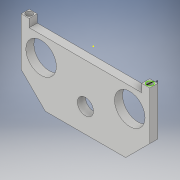
# Autodesk Inventor part: Middle_part
Saved by Autodesk Inventor 2019 (Build 230136000, 136)
## iProperties
Created: 2021-06-20
Part Number: Middle_part
Material: Generic
Document SubType Name: Modeling
Designer: 91742
Density: 1 g/cm^3
Appearance: Default
Author: 91742
Autodesk Inventor part; units mm, degrees
ref_plane "YZ Plane" through (0, 0, 0) normal (1, 0, 0) x (0, 1, 0)
ref_plane "XZ Plane" through (0, 0, 0) normal (0, 1, 0) x (-1, 0, 0)
ref_plane "XY Plane" through (0, 0, 0) normal (0, 0, 1) x (1, 0, 0)
sketch "Sketch1" plane through (0, 0, 0) normal (0, 0, 1) x (1, 0, 0)
  line L0 (-40, 5) -> (40, 5)
  circle A0 centre (-27.6, 32.5) radius 9.5
  line L1 (-40, 5) -> (-40, 50)
  line L2 (-40, 50) -> (-35, 50)
  line L3 (-35, 50) -> (-35, 45)
  line L4 (-35, 45) -> (0, 45)
  circle A1 centre (27.6, 32.5) radius 9.5
  line L5 (40, 5) -> (40, 50)
  line L6 (40, 50) -> (35, 50)
  line L7 (35, 50) -> (35, 45)
  line L8 (35, 45) -> (0, 45)
  circle A2 centre (0, 20) radius 5
  point P0 (0, 0)
  dimension "d0" = 80
  dimension "d3" = 19
  dimension "d4" = 45
  dimension "d5" = 5
  dimension "d6" = 5
  dimension "d7" = 10
  constraints: 18 end point, 3 centre point, 3 perpendicular, 1 horizontal, 1 vertical
  measures "d0" distance of L0.start L0.end
  measures "d3" diameter of A0
  measures "d4" distance of L0.start L1.end
  measures "d5" distance of L1.end L2.end
  measures "d6" distance of L2.end L3.end
  measures "d7" diameter of A2
extrude "Extrusion1" add sketch "Sketch1" along normal blind 5
chamfer "Chamfer1" distance 15 angle 45 2 edges at (40, 5, 2.5) (-40, 5, 2.5)
sketch "Sketch3" plane through (35, 50, 0) normal (0, 1, 0) x (1, 0, 0)
  circle A0 centre (2.5, -2.5) radius 2
  point P0 (-35, 0)
  dimension "d13" = 4
  constraints: 1 centre point
  measures "d13" diameter of A0
sketch "Sketch4" plane through (-40, 50, 0) normal (0, 1, 0) x (1, 0, 0)
  circle A0 centre (2.5, -2.5) radius 2
  point P0 (40, 0)
  dimension "d14" = 4
  constraints: 1 centre point
  measures "d14" diameter of A0
hole "Hole1" at (-37.5, 50, 2.5) direction (0, -1, 0) diameter 4 depth 4
hole "Hole2" at (37.5, 50, 2.5) direction (0, -1, 0) diameter 4 depth 4
body "Solid1"
